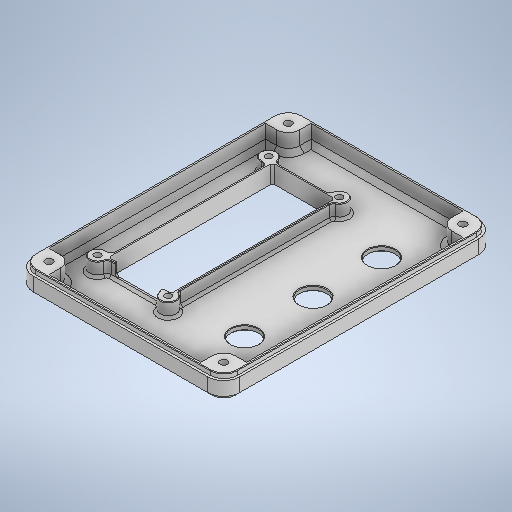
# Autodesk Inventor part: PCB-HousingBottom
Saved by Autodesk Inventor 2025.1 (Build 291241000, 241)
## iProperties
Created: 2025-03-29
Part Number: PCB-HousingBottom
Material: Všeobecné
Document SubType Name: Modeling
Designer: 42060
Density: 1 g/cm^3
Appearance: Výchozí
Author: 42060
Autodesk Inventor part; units mm, degrees
(part 1 of 4)
ref_plane "YZ Plane" through (0, 0, 0) normal (1, 0, 0) x (0, 1, 0)
ref_plane "XZ Plane" through (0, 0, 0) normal (0, 1, 0) x (-1, 0, 0)
ref_plane "XY Plane" through (0, 0, 0) normal (0, 0, 1) x (1, 0, 0)
sketch "Náčrt1" plane through (0, 0, 0) normal (0, 1, 0) x (-1, 0, 0)
  circle A0 centre (37.7, 43.65) radius 1.6
  circle A1 centre (-19.7, 43.65) radius 1.6
  arc A2 (41.3, 43.65) -> (37.7, 47.25) centre (37.7, 43.65) ccw
  arc A3 (-19.7, 47.25) -> (-23.3, 43.65) centre (-19.7, 43.65) ccw
  line L0 (38.3, 57.45) -> (-38.3, 57.45)
  line L1 (37.7, 47.25) -> (-19.7, 47.25)
  line L2 (-43.3, 52.45) -> (-43.3, -52.45)
  line L3 (-43.3, 57.45) -> (43.3, -57.45) construction
  line L4 (43.3, 57.45) -> (-43.3, -57.45) construction
  line L5 (43.3, -52.45) -> (43.3, 52.45)
  line L6 (41.3, -43.65) -> (41.3, 43.65)
  line L7 (-23.3, 43.65) -> (-23.3, -43.65)
  line L8 (41.3, 47.25) -> (-23.3, -47.25) construction
  line L9 (-23.3, 47.25) -> (41.3, -47.25) construction
  line L10 (-38.3, -57.45) -> (38.3, -57.45)
  circle A4 centre (37.7, -43.65) radius 1.6
  arc A5 (37.7, -47.25) -> (41.3, -43.65) centre (37.7, -43.65) ccw
  circle A6 centre (-19.7, -43.65) radius 1.6
  line L11 (-19.7, -47.25) -> (37.7, -47.25)
  arc A7 (-23.3, -43.65) -> (-19.7, -47.25) centre (-19.7, -43.65) ccw
  arc A8 (43.3, 52.45) -> (38.3, 57.45) centre (38.3, 52.45) ccw
  arc A9 (38.3, -57.45) -> (43.3, -52.45) centre (38.3, -52.45) ccw
  arc A10 (-43.3, -52.45) -> (-38.3, -57.45) centre (-38.3, -52.45) ccw
  arc A11 (-38.3, 57.45) -> (-43.3, 52.45) centre (-38.3, 52.45) ccw
  line L12 (45.3, 52.45) -> (45.3, -52.45)
  arc A12 (38.3, -59.45) -> (45.3, -52.45) centre (38.3, -52.45) ccw
  line L13 (38.3, -59.45) -> (-38.3, -59.45)
  arc A13 (-45.3, -52.45) -> (-38.3, -59.45) centre (-38.3, -52.45) ccw
  line L14 (-45.3, -52.45) -> (-45.3, 52.45)
  arc A14 (-38.3, 59.45) -> (-45.3, 52.45) centre (-38.3, 52.45) ccw
  line L15 (-38.3, 59.45) -> (38.3, 59.45)
  arc A15 (45.3, 52.45) -> (38.3, 59.45) centre (38.3, 52.45) ccw
  circle A16 centre (-38.3, 52.45) radius 1.625
  circle A17 centre (-38.3, 52.45) radius 5
  line L16 (-38.3, 47.45) -> (-43.3, 47.45)
  line L17 (-33.3, 52.45) -> (-33.3, 57.45)
  line L18 (43.3, 0) -> (-43.3, 0)
  line L19 (0, 57.45) -> (0, -57.45)
  circle A18 centre (-38.3, -52.45) radius 1.625
  circle A19 centre (-38.3, -52.45) radius 5
  line L20 (-38.3, -47.45) -> (-43.3, -47.45)
  line L21 (-33.3, -52.45) -> (-33.3, -57.45)
  circle A20 centre (38.3, 52.45) radius 5
  circle A21 centre (38.3, 52.45) radius 1.625
  line L22 (33.3, 52.45) -> (33.3, 57.45)
  circle A22 centre (38.3, -52.45) radius 5
  circle A23 centre (38.3, -52.45) radius 1.625
  line L23 (33.3, -52.45) -> (33.3, -57.45)
  line L24 (38.3, -47.45) -> (43.3, -47.45)
  line L25 (38.3, 47.45) -> (43.3, 47.45)
  point P0 (0, 0)
  point P1 (0, 0)
  point P2 (0, 0)
  point P3 (-43.3, -47.45)
  point P4 (-33.3, -57.45)
  point P5 (39.783171, -46.586051)
  point P6 (39.099517, -45.78373)
  point P7 (39.783171, 49.186051)
  point P8 (39.099517, 45.78373)
  point P9 (43.3, -52.45)
  point P10 (38.3, -57.45)
  point P11 (43.3, -52.45)
  point P12 (38.3, -57.45)
  dimension "d0" = 94.5
  dimension "d1" = 64.6
  dimension "d2" = 3.2
  dimension "d3" = 3.6
  dimension "d4" = 3.6
  dimension "d5" = 3.6
  dimension "d6" = 3.6
  dimension "d7" = 3.6
  dimension "d10" = 2
  dimension "d11" = 10.2
  dimension "d12" = 20
  dimension "d13" = 10.2
  dimension "d14" = 5
  dimension "d15" = 2
  dimension "d59" = 3.25
  constraints: 52 end point, 32 point on circle, 24 centre point, 21 point on line, 21 tangent, 12 equal radius, 10 symmetric about line, 8 coincident, 6 midpoint, 6 parallel, 5 perpendicular, 4 horizontal, 2 horizontal alignment, 2 vertical alignment, 1 vertical, 11 other
  measures "d0" distance of L9.end L8.start
  measures "d1" distance of L8.end L9.end
  measures "d2" diameter of A0
  measures "d3" distance from line of L6 A0.centre
  measures "d4" distance from line of L1 A0.centre
  measures "d5" distance from line of L7 A1.centre
  measures "d6" distance from line of L11 A4.centre
  measures "d7" radius of A3
  measures "d10" distance between parallel lines of L5 L6
  measures "d11" distance between parallel lines of L10 L11
  measures "d12" distance between parallel lines of L2 L7
  measures "d13" distance between parallel lines of L0 L1
  measures "d14" radius of A8
  measures "d15" distance between parallel lines of L5 L12
  measures "d59" diameter of A16
extrude "Vysunutí1" add sketch "Náčrt1" against normal blind 2 contours A0 | A1 | L6 L18 L19 L1 A2 | A2 L1 L19 L0 L22 A20 L25 L5 L18 L6 | L18 L5 L24 A22 L23 L10 L19 L11 A5 L6 | L6 A5 L11 L19 L18 | L19 L18 L7 A3 L1 | L1 A3 L7 L18 L2 L16 A17 L17 L0 L19 | L19 L11 A7 L7 L18 | L5 A22 L24 | L25 A20 L5 | L7 A7 L11 L19 L10 L21 A19 L20 L2 L18 | L0 A20 L22 | L17 A17 L0 | A9 A22 | A20 A8 | A17 A11 | L10 L23 A22 | L2 A17 L16 | L20 A19 L2 | L10 A19 L21 | A19 A10 | A4 | A6 | L12 A12 L13 A13 L14 A14 L15 A15
extrude "Vysunutí2" add sketch "Náčrt1" along normal blind 8 contours L5 A22 L24 | L25 A20 L5 | L0 A20 L22 | L17 A17 L0 | A9 A22 | A20 A8 | A17 A11 | L10 L23 A22 | L2 A17 L16 | L20 A19 L2 | L10 A19 L21 | A19 A10 | L12 A12 L13 A13 L14 A14 L15 A15
sketch "Náčrt2" plane through (0, 0, 0) normal (0, -1, 0) x (1, 0, 0)
  circle A0 centre (25, -30) radius 6
  circle A1 centre (25, 0) radius 6
  circle A2 centre (25, 30) radius 6
  line L0 (-28.4, -35.65) -> (-1.6, -35.65)
  line L1 (-1.6, -35.65) -> (-1.6, 35.65)
  line L2 (-1.6, 35.65) -> (-28.4, 35.65)
  line L3 (-28.4, 35.65) -> (-28.4, -35.65)
  line L4 (-28.4, -35.65) -> (-1.6, 35.65) construction
  line L5 (-1.6, -35.65) -> (-28.4, 35.65) construction
  line L6 (25, -30) -> (25, 0) construction
  line L7 (25, 0) -> (25, 30) construction
  circle A3 centre (-32, 37.5) radius 1.45
  circle A4 centre (-32, -37.5) radius 1.45
  circle A5 centre (-1, -37.5) radius 1.45
  circle A6 centre (-1, 37.5) radius 1.45
  line L8 (-28.7, -35.95) -> (-1.3, -35.95)
  line L9 (-1.3, -35.95) -> (-1.3, 35.95)
  line L10 (-1.3, 35.95) -> (-28.7, 35.95)
  line L11 (-28.7, 35.95) -> (-28.7, -35.95)
  arc A7 (-31.681818, -34.014493) -> (-28.591591, -38.295455) centre (-32, -37.5) ccw
  arc A8 (-28.591591, 38.295455) -> (-31.681818, 34.014493) centre (-32, 37.5) ccw
  line L12 (-6.356071, -36.75) -> (-26.643929, -36.75)
  line L13 (-29.5, -32.022774) -> (-29.5, 32.022774)
  line L14 (-26.643929, 36.75) -> (-6.356071, 36.75)
  line L15 (-0.5, 32.601021) -> (-0.5, -32.601021)
  arc A9 (-4.408409, -38.295455) -> (-6.356071, -36.75) centre (-6.356071, -38.75) ccw
  arc A10 (-0.5, -32.601021) -> (0.590909, -34.382468) centre (1.5, -32.601021) ccw
  arc A11 (0.590909, 34.382468) -> (-0.5, 32.601021) centre (1.5, 32.601021) ccw
  arc A12 (-6.356071, 36.75) -> (-4.408409, 38.295455) centre (-6.356071, 38.75) ccw
  arc A13 (-28.591591, 38.295455) -> (-26.643929, 36.75) centre (-26.643929, 38.75) ccw
  arc A14 (-29.5, 32.022774) -> (-31.681818, 34.014493) centre (-31.5, 32.022774) ccw
  arc A15 (-31.681818, -34.014493) -> (-29.5, -32.022774) centre (-31.5, -32.022774) ccw
  arc A16 (-26.643929, -36.75) -> (-28.591591, -38.295455) centre (-26.643929, -38.75) ccw
  arc A17 (-4.408409, -38.295455) -> (0.590909, -34.382468) centre (-1, -37.5) ccw
  arc A18 (0.590909, 34.382468) -> (-4.408409, 38.295455) centre (-1, 37.5) ccw
  line L16 (-29.5, -33.25) -> (-28.4, -33.25)
  arc A19 (-29.5, -33.25) -> (-30.15522, -33.503169) centre (-29.5, -34.224465) ccw
  line L17 (-29.5, 7.3) -> (-28.4, 7.3)
  line L18 (-25, 36.75) -> (-25, 35.65)
  line L19 (-5, 36.75) -> (-5, 35.65)
  arc A20 (-4.73177, 37.583104) -> (-5, 36.75) centre (-3.572102, 36.75) ccw
  point P0 (0, 0)
  point P1 (-15, 0)
  point P2 (-28.7, -33.25)
  point P3 (-28.7, 7.3)
  point P4 (-15, 35.65)
  point P5 (-5, 35.95)
  point P6 (-25, 35.95)
  dimension "d23" = 71.3
  dimension "d24" = 26.8
  dimension "d25" = 12
  dimension "d26" = 2.9
  dimension "d27" = 75
  dimension "d28" = 31
  dimension "d30" = 1.85
  dimension "d31" = 3.6
  dimension "d32" = 0.3
  dimension "d33" = 30
  dimension "d34" = 15
  dimension "d35" = 25
  dimension "d39" = 0.8
  dimension "d40" = 0.8
  dimension "d41" = 0.8
  dimension "d42" = 0.8
  dimension "d43" = 2
  dimension "d44" = 3.5
  dimension "d47" = 2.4
  dimension "d48" = 40.55
  dimension "d49" = 10
  dimension "d50" = 20
  constraints: 40 end point, 30 point on circle, 21 centre point, 20 tangent, 15 equal radius, 8 point on line, 6 parallel, 6 perpendicular, 4 coincident, 4 horizontal alignment, 4 vertical alignment, 3 horizontal, 3 midpoint, 2 collinear, 1 vertical, 3 other
  measures "d23" distance of L2.end L0.start
  measures "d24" distance between parallel lines of L1 L3
  measures "d25" diameter of A0
  measures "d26" diameter of A3
  measures "d27" distance of A4.centre A3.centre
  measures "d28" distance of A6.centre A3.centre
  measures "d30" distance from line of A3.centre L2
  measures "d31" distance from line of L3 A3.centre
  measures "d32" distance between parallel lines of L3 L11
  measures "d33" distance of L6.end L7.end
  measures "d34" distance of point (0, 0) point (-15, 0)
  measures "d35" distance of L6.end point (0, 0)
  measures "d39" distance between parallel lines of L8 L12
  measures "d40" distance between parallel lines of L11 L13
  measures "d41" distance between parallel lines of L10 L14
  measures "d42" distance between parallel lines of L9 L15
  measures "d43" radius of A9
  measures "d44" radius of A17
  measures "d47" distance between parallel lines of L0 L16
  measures "d48" distance between parallel lines of L16 L17
  measures "d49" distance from line of point (-15, 35.65) L18
  measures "d50" distance between parallel lines of L19 L18
extrude "Vysunutí4" cut sketch "Náčrt2" along normal through all contours A0 | A1 | A2 | L3 L2 L1 L0 | L0 L1 L2 L19 L10 L9 L8 L11 L16 L3 | L16 L11 L17 L3 | L17 L11 L10 L18 L2 L3 | L2 L18 L10 L19
extrude "Vysunutí5" add sketch "Náčrt2" against normal blind 6.1 contours L16 A19 A15 L13 L17 L11 | L11 L8 L9 L10 L19 A20 A12 A18 A11 L15 A10 A17 A9 L12 A16 A7 A15 A19 L16 | L17 L13 A14 A8 A13 L14 L18 L10 L11
extrude "Vysunutí6" add sketch "Náčrt2" against normal blind 1 contours L10 L18 L14 A12 A20 L19
chamfer "Zkosení1" distance 1 angle 45 3 edges at (-25, 1, 36.35) (-5, 1, 36.35) (-4.9313, 1, 37.1876)
sketch "Náčrt3" plane through (0, 8, 0) normal (0, 1, 0) x (1, 0, 0)
  line L0 (45.3, -52.45) -> (45.3, 52.45) projected
  arc A0 (45.3, 52.45) -> (38.3, 59.45) centre (38.3, 52.45) ccw projected
  line L1 (38.3, 59.45) -> (-38.3, 59.45) projected
  arc A1 (-38.3, 59.45) -> (-45.3, 52.45) centre (-38.3, 52.45) ccw projected
  line L2 (-45.3, 52.45) -> (-45.3, -52.45) projected
  arc A2 (-45.3, -52.45) -> (-38.3, -59.45) centre (-38.3, -52.45) ccw projected
  line L3 (-38.3, -59.45) -> (38.3, -59.45) projected
  arc A3 (38.3, -59.45) -> (45.3, -52.45) centre (38.3, -52.45) ccw projected
  line L4 (-33.3, 57.45) -> (33.3, 57.45) projected
  line L5 (43.3, 47.45) -> (43.3, -47.45) projected
  line L6 (33.3, -57.45) -> (-33.3, -57.45) projected
  line L7 (-43.3, -47.45) -> (-43.3, 47.45) projected
  line L8 (33.3, 57.45) -> (33.3, 52.45) projected
  arc A4 (33.3, 52.45) -> (38.3, 47.45) centre (38.3, 52.45) ccw projected
  line L9 (38.3, 47.45) -> (43.3, 47.45) projected
  line L10 (43.3, -47.45) -> (38.3, -47.45) projected
  arc A5 (38.3, -47.45) -> (33.3, -52.45) centre (38.3, -52.45) ccw projected
  line L11 (33.3, -52.45) -> (33.3, -57.45) projected
  line L12 (-38.3, 58.4) -> (38.3, 58.4)
  arc A6 (44.25, 52.45) -> (38.3, 58.4) centre (38.3, 52.45) ccw
  line L13 (44.25, 52.45) -> (44.25, -52.45)
  arc A7 (38.3, -58.4) -> (44.25, -52.45) centre (38.3, -52.45) ccw
  line L14 (38.3, -58.4) -> (-38.3, -58.4)
  arc A8 (-44.25, -52.45) -> (-38.3, -58.4) centre (-38.3, -52.45) ccw
  line L15 (-44.25, -52.45) -> (-44.25, 52.45)
  arc A9 (-38.3, 58.4) -> (-44.25, 52.45) centre (-38.3, 52.45) ccw
  line L16 (-43.3, 47.45) -> (-38.3, 47.45) projected
  arc A10 (-38.3, 47.45) -> (-33.3, 52.45) centre (-38.3, 52.45) ccw projected
  line L17 (-33.3, 52.45) -> (-33.3, 57.45) projected
  line L18 (-33.3, -57.45) -> (-33.3, -52.45) projected
  arc A11 (-33.3, -52.45) -> (-38.3, -47.45) centre (-38.3, -52.45) ccw projected
  line L19 (-38.3, -47.45) -> (-43.3, -47.45) projected
  point P0 (0, 0)
  dimension "d67" = 1.05
  constraints: 8 end point, 8 point on circle, 4 centre point, 7 other
  measures "d67" distance between parallel lines of L1 L12
extrude "Vysunutí7" cut sketch "Náčrt3" against normal blind 2 contours A3 L3 A2 L2 A1 L1 A0 L0
sketch "Náčrt4" plane through (0, -2, 0) normal (0, -1, 0) x (1, 0, 0)
  circle A0 centre (-38.3, -52.45) radius 1.625 projected
  circle A1 centre (-38.3, 52.45) radius 1.625 projected
  circle A2 centre (38.3, 52.45) radius 1.625 projected
  circle A3 centre (38.3, -52.45) radius 1.625 projected
  point P0 (0, 0)
  constraints: 4 coincident
hole "Díra1" at (-38.3, -2, -52.45) at (-38.3, -2, 52.45) at (38.3, -2, 52.45) at (38.3, -2, -52.45) direction (0, 1, 0) diameter 5.7 depth 3
chamfer "Zkosení3" distance 2 angle 45 24 edges at (34.7645, 0, -48.9145) (33.3, 0, -54.95) (40.8, 0, -47.45) (43.3, 0, 0) (33.3, 0, 54.95) (34.7645, 0, 48.9145) (40.8, 0, 47.45) (0, 0, 57.45) (-34.7645, 0, 48.9145) (-33.3, 0, 54.95) (-40.8, 0, 47.45) (-43.3, 0, 0) (-33.3, 0, -54.95) (-34.7645, 0, -48.9145) (-40.8, 0, -47.45) (0, 0, -57.45) (0, -2, -59.45) (43.2497, -2, -57.3997) (45.3, -2, 0) (43.2497, -2, 57.3997) (0, -2, 59.45) (-43.2497, -2, 57.3997) (-45.3, -2, 0) (-43.2497, -2, -57.3997)
chamfer "Zkosení5" distance 1 angle 45 20 edges at (-1.3, 2.05, 35.95) (-1.3, 2.05, -35.95) (-28.7, 2.05, -35.95) (-28.7, 2.05, 35.95) (-16.5, 0, 36.75) (-27.8871, 0, 37.1833) (-34.8379, 0, 39.5485) (-30.1516, 0, 33.4999) (-29.5, 0, 0) (-30.1516, 0, -33.4999) (-34.8379, 0, -39.5485) (-27.8871, 0, -37.1833) (-16.5, 0, -36.75) (-5.1129, 0, -37.1833) (1.1572, 0, -40.2561) (-0.2056, 0, -33.6455) (-0.5, 0, 0) (-0.2056, 0, 33.6455) (1.1572, 0, 40.2561) (-5.1129, 0, 37.1833)
chamfer "Zkosení2" distance 0.25 angle 45 44 edges at (-44.25, 8, 0) (-42.5073, 8, 56.6573) (0, 8, 58.4) (42.5073, 8, 56.6573) (44.25, 8, 0) (42.5073, 8, -56.6573) (0, 8, -58.4) (-42.5073, 8, -56.6573) (19, 0, -30) (19, -2, -30) (19, 0, 0) (19, -2, 0) (19, 0, 30) (19, -2, 30) (-1.3, -2, 0) (-15, -2, -35.95) (-28.7, -2, 0) (-15, -2, 35.95) (38.3, -2, 55.3) (38.3, -2, -49.6) (-38.3, -2, -49.6) (-38.3, -2, 55.3) (-27.8871, 6.1, 37.1833) (-25.822, 6.1, 36.75) (-34.8379, 6.1, 39.5485) (-30.1516, 6.1, 33.4999) (-29.5, 6.1, 0) (-30.1516, 6.1, -33.4999) (-34.8379, 6.1, -39.5485) (-27.8871, 6.1, -37.1833) (-16.5, 6.1, -36.75) (-5.1129, 6.1, -37.1833) (1.1572, 6.1, -40.2561) (-0.2056, 6.1, -33.6455) (-0.5, 6.1, 0) (-0.2056, 6.1, 33.6455) (1.1572, 6.1, 40.2561) (-4.5349, 6.1, 37.9233) (-4.9313, 6.1, 37.1876) (-5, 6.1, 36.35) (-28.2001, -2, -35.45) (-28.2, -2, 35.45) (-1.8, -2, 35.4501) (-1.8, -2, -35.45)
sketch "Náčrt5" plane through (0, -2, 0) normal (0, -1, 0) x (1, 0, 0)
  line L0 (3.529017, -37.317035) -> (3.529017, -22.682965) construction
  line L1 (3.529017, -22.682965) -> (6.470983, -22.682965) construction
  line L2 (6.470983, -22.682965) -> (6.470983, -37.317035) construction
  line L3 (6.470983, -37.317035) -> (3.529017, -37.317035) construction
  line L4 (3.529017, -8.753762) -> (3.529017, 8.753762) construction
  line L5 (3.529017, 8.753762) -> (6.470983, 8.753762) construction
  line L6 (6.470983, 8.753762) -> (6.470983, -8.753762) construction
  line L7 (6.470983, -8.753762) -> (3.529017, -8.753762) construction
  line L8 (3.529017, 19.285961) -> (3.529017, 40.714039) construction
  line L9 (3.529017, 40.714039) -> (6.470983, 40.714039) construction
  line L10 (6.470983, 40.714039) -> (6.470983, 19.285961) construction
  line L11 (6.470983, 19.285961) -> (3.529017, 19.285961) construction
  circle A0 centre (25, -30) radius 6.25
  circle A1 centre (25, 0) radius 6.25
  circle A2 centre (25, 30) radius 6.25
  line L12 (-40.028603, -44.09129) -> (-40.028603, 44.09129) construction
  line L13 (-40.028603, 44.09129) -> (-36.91312, 44.09129) construction
  line L14 (-36.91312, 44.09129) -> (-36.91312, -44.09129) construction
  line L15 (-36.91312, -44.09129) -> (-40.028603, -44.09129) construction
  line L16 (-43.3, -52.45) -> (-43.3, 52.45)
  line L17 (3.534054, -35.342469) -> (3.534054, -34.612081)
  line L18 (3.534054, -34.612081) -> (9.634054, -32.748332)
  line L19 (9.634054, -32.748332) -> (9.634054, -33.760801)
  line L20 (9.634054, -33.760801) -> (5.150982, -34.974756)
  line L21 (5.150982, -34.974756) -> (9.634054, -36.188712)
  line L22 (9.634054, -36.188712) -> (9.634054, -37.206218)
  line L23 (9.634054, -37.206218) -> (3.534054, -35.342469)
  line L24 (7.573856, -36.188712) -> (7.573856, -33.715466)
  line L25 (7.573856, -33.715466) -> (8.485582, -33.715466)
  line L26 (8.485582, -33.715466) -> (8.485582, -36.188712)
  line L27 (8.485582, -36.188712) -> (7.573856, -36.188712)
  line L28 (6.163451, -31.660305) -> (6.163451, -30.053451)
  spline S0 degree 2 poles (6.163451, -30.053451) (6.163451, -29.857002) (6.002262, -29.574921) (5.689958, -29.418769) (5.478397, -29.418769) knots 0 0 0 1 2 3 3 3
  line L29 (5.478397, -29.418769) -> (5.150982, -29.418769)
  spline S1 degree 2 poles (5.150982, -29.418769) (4.939421, -29.418769) (4.62208, -29.574921) (4.44578, -29.857002) (4.44578, -30.053451) knots 0 0 0 1 2 3 3 3
  line L30 (4.44578, -30.053451) -> (4.44578, -31.660305)
  line L31 (4.44578, -31.660305) -> (3.529017, -31.660305)
  line L32 (3.529017, -31.660305) -> (3.529017, -30.0736)
  spline S2 degree 2 poles (3.529017, -30.0736) (3.529017, -29.569884) (3.911841, -28.824385) (4.632155, -28.426449) (5.120759, -28.426449) knots 0 0 0 1 2 3 3 3
  line L33 (5.120759, -28.426449) -> (5.47336, -28.426449)
  spline S3 degree 2 poles (5.47336, -28.426449) (5.967002, -28.426449) (6.692353, -28.824385) (7.085251, -29.569884) (7.085251, -30.0736) knots 0 0 0 1 2 3 3 3
  line L34 (7.085251, -30.0736) -> (7.085251, -31.660305)
  line L35 (7.085251, -31.660305) -> (6.163451, -31.660305)
  line L36 (3.529017, -32.07839) -> (3.529017, -31.121329)
  line L37 (3.529017, -31.121329) -> (9.634054, -31.121329)
  line L38 (9.634054, -31.121329) -> (9.634054, -32.07839)
  line L39 (9.634054, -32.07839) -> (3.529017, -32.07839)
  line L40 (6.893839, -30.451387) -> (6.702427, -29.504401)
  line L41 (6.702427, -29.504401) -> (9.634054, -28.214888)
  line L42 (9.634054, -28.214888) -> (9.634054, -29.312989)
  line L43 (9.634054, -29.312989) -> (6.893839, -30.451387)
  line L44 (9.719474, -22.556254) -> (9.719474, -23.249664)
  line L45 (9.719474, -23.249664) -> (5.036443, -23.249664)
  line L46 (5.036443, -23.249664) -> (8.242209, -24.852547)
  line L47 (8.242209, -24.852547) -> (5.036443, -26.45543)
  line L48 (5.036443, -26.45543) -> (9.719474, -26.45543)
  line L49 (9.719474, -26.45543) -> (9.719474, -27.14884)
  line L50 (9.719474, -27.14884) -> (3.619474, -27.14884)
  line L51 (3.619474, -27.14884) -> (3.619474, -26.555924)
  line L52 (3.619474, -26.555924) -> (6.955883, -24.852547)
  line L53 (6.955883, -24.852547) -> (3.619474, -23.149169)
  line L54 (3.619474, -23.149169) -> (3.619474, -22.556254)
  line L55 (3.619474, -22.556254) -> (9.719474, -22.556254)
  spline S4 degree 2 poles (9.754946, -6.537412) (9.754946, -7.03609) (9.457753, -7.806776) (8.868405, -8.315529) (8.43521, -8.416272) knots 0 0 0 1 2 3 3 3
  line L56 (8.43521, -8.416272) -> (8.037274, -7.509583)
  spline S5 degree 2 poles (8.037274, -7.509583) (8.425135, -7.398766) (8.828108, -6.879939) (8.828108, -6.502152) knots 0 0 0 1 2 2 2
  spline S6 degree 2 poles (8.828108, -6.502152) (8.828108, -6.07903) (8.455358, -5.605537) (8.122906, -5.605537) knots 0 0 0 1 2 2 2
  line L57 (8.122906, -5.605537) -> (7.850899, -5.605537)
  spline S7 degree 2 poles (7.850899, -5.605537) (7.614153, -5.605537) (7.306886, -5.867469) (7.135623, -6.270442) (7.034879, -6.602895) knots 0 0 0 1 2 3 3 3
  spline S8 degree 2 poles (7.034879, -6.602895) (7.029842, -6.607932) (7.024805, -6.628081) (7.019768, -6.638155) knots 0 0 0 1 2 2 2
  line L58 (7.019768, -6.638155) -> (7.009694, -6.683489)
  spline S9 degree 2 poles (7.009694, -6.683489) (6.863616, -7.187205) (6.556349, -7.821887) (5.896481, -8.270195) (5.337357, -8.270195) knots 0 0 0 1 2 3 3 3
  line L59 (5.337357, -8.270195) -> (5.17113, -8.270195)
  spline S10 degree 2 poles (5.17113, -8.270195) (4.652303, -8.270195) (3.911841, -7.836999) (3.529016, -7.005868) (3.529016, -6.421557) knots 0 0 0 1 2 3 3 3
  spline S11 degree 2 poles (3.529016, -6.421557) (3.529016, -5.978287) (3.821172, -5.29827) (4.385334, -4.839889) (4.803418, -4.729071) knots 0 0 0 1 2 3 3 3
  line L60 (4.803418, -4.729071) -> (5.206391, -5.6005)
  spline S12 degree 2 poles (5.206391, -5.6005) (4.838678, -5.711318) (4.455854, -6.154588) (4.455854, -6.45178) knots 0 0 0 1 2 2 2
  spline S13 degree 2 poles (4.455854, -6.45178) (4.455854, -6.864827) (4.808455, -7.313134) (5.130833, -7.313134) knots 0 0 0 1 2 2 2
  line L61 (5.130833, -7.313134) -> (5.33232, -7.313134)
  spline S14 degree 2 poles (5.33232, -7.313134) (5.584178, -7.313134) (5.891444, -7.046165) (6.067745, -6.638155) (6.173525, -6.280517) knots 0 0 0 1 2 3 3 3
  spline S15 degree 2 poles (6.173525, -6.280517) (6.183599, -6.260368) (6.193674, -6.220071) (6.203748, -6.194885) knots 0 0 0 1 2 2 2
  spline S16 degree 2 poles (6.203748, -6.194885) (6.208785, -6.179773) (6.21886, -6.139476) (6.223897, -6.119327) knots 0 0 0 1 2 2 2
  spline S17 degree 2 poles (6.223897, -6.119327) (6.364937, -5.660946) (6.682278, -5.061524) (7.31696, -4.653514) (7.845862, -4.653514) knots 0 0 0 1 2 3 3 3
  line L62 (7.845862, -4.653514) -> (8.117869, -4.653514)
  spline S18 degree 2 poles (8.117869, -4.653514) (8.636696, -4.653514) (9.372121, -5.096784) (9.754946, -5.943027) (9.754946, -6.537412) knots 0 0 0 1 2 3 3 3
  line L63 (4.098215, -2.961028) -> (4.098215, -1.998931)
  line L64 (4.098215, -1.998931) -> (9.6945, -1.998931)
  line L65 (9.6945, -1.998931) -> (9.6945, -2.961028)
  line L66 (9.6945, -2.961028) -> (4.098215, -2.961028)
  line L67 (3.5945, -4.331136) -> (3.5945, -0.628824)
  line L68 (3.5945, -0.628824) -> (4.511263, -0.628824)
  line L69 (4.511263, -0.628824) -> (4.511263, -4.331136)
  line L70 (4.511263, -4.331136) -> (3.5945, -4.331136)
  spline S19 degree 2 poles (9.754946, 1.647973) (9.754946, 1.083811) (9.306638, 0.237568) (8.460396, -0.215777) (7.891197, -0.215777) knots 0 0 0 1 2 3 3 3
  line L71 (7.891197, -0.215777) -> (5.397803, -0.215777)
  spline S20 degree 2 poles (5.397803, -0.215777) (4.828604, -0.215777) (3.982361, 0.237568) (3.529016, 1.083811) (3.529016, 1.647973) knots 0 0 0 1 2 3 3 3
  spline S21 degree 2 poles (3.529016, 1.647973) (3.529016, 2.217172) (3.982361, 3.058377) (4.828604, 3.511722) (5.397803, 3.511722) knots 0 0 0 1 2 3 3 3
  line L72 (5.397803, 3.511722) -> (7.891197, 3.511722)
  spline S22 degree 2 poles (7.891197, 3.511722) (8.460396, 3.511722) (9.306638, 3.058377) (9.754946, 2.217172) (9.754946, 1.647973) knots 0 0 0 1 2 3 3 3
  spline S23 degree 2 poles (8.802922, 1.647973) (8.802922, 1.919979) (8.57625, 2.317915) (8.158166, 2.529475) (7.876085, 2.529475) knots 0 0 0 1 2 3 3 3
  line L73 (7.876085, 2.529475) -> (5.407877, 2.529475)
  spline S24 degree 2 poles (5.407877, 2.529475) (5.125796, 2.529475) (4.707712, 2.317915) (4.48104, 1.919979) (4.48104, 1.647973) knots 0 0 0 1 2 3 3 3
  spline S25 degree 2 poles (4.48104, 1.647973) (4.48104, 1.381003) (4.707712, 0.983067) (5.125796, 0.76647) (5.407877, 0.76647) knots 0 0 0 1 2 3 3 3
  line L74 (5.407877, 0.76647) -> (7.876085, 0.76647)
  spline S26 degree 2 poles (7.876085, 0.76647) (8.158166, 0.76647) (8.57625, 0.983067) (8.802922, 1.381003) (8.802922, 1.647973) knots 0 0 0 1 2 3 3 3
  line L75 (6.410272, 5.032944) -> (6.410272, 6.569277)
  spline S27 degree 2 poles (6.410272, 6.569277) (6.410272, 6.760689) (6.228934, 7.052845) (5.896481, 7.208997) (5.674846, 7.208997) knots 0 0 0 1 2 3 3 3
  line L76 (5.674846, 7.208997) -> (5.261799, 7.208997)
  spline S28 degree 2 poles (5.261799, 7.208997) (5.035127, 7.208997) (4.6926, 7.052845) (4.511263, 6.760689) (4.511263, 6.569277) knots 0 0 0 1 2 3 3 3
  line L77 (4.511263, 6.569277) -> (4.511263, 5.032944)
  line L78 (4.511263, 5.032944) -> (3.5945, 5.032944)
  line L79 (3.5945, 5.032944) -> (3.5945, 6.554166)
  spline S29 degree 2 poles (3.5945, 6.554166) (3.5945, 7.057882) (3.987398, 7.793307) (4.722823, 8.191243) (5.221502, 8.191243) knots 0 0 0 1 2 3 3 3
  line L80 (5.221502, 8.191243) -> (5.720181, 8.191243)
  spline S30 degree 2 poles (5.720181, 8.191243) (6.213822, 8.191243) (6.939173, 7.793307) (7.327035, 7.057882) (7.327035, 6.554166) knots 0 0 0 1 2 3 3 3
  line L81 (7.327035, 6.554166) -> (7.327035, 5.032944)
  line L82 (7.327035, 5.032944) -> (6.410272, 5.032944)
  line L83 (3.5945, 4.559451) -> (3.5945, 5.521548)
  line L84 (3.5945, 5.521548) -> (9.6945, 5.521548)
  line L85 (9.6945, 5.521548) -> (9.6945, 4.559451)
  line L86 (9.6945, 4.559451) -> (3.5945, 4.559451)
  line L87 (6.223897, 20.258133) -> (6.223897, 21.864987)
  spline S31 degree 2 poles (6.223897, 21.864987) (6.223897, 22.061436) (6.062708, 22.343517) (5.750404, 22.499669) (5.538843, 22.499669) knots 0 0 0 1 2 3 3 3
  line L88 (5.538843, 22.499669) -> (5.211428, 22.499669)
  spline S32 degree 2 poles (5.211428, 22.499669) (4.999867, 22.499669) (4.682526, 22.343517) (4.506225, 22.061436) (4.506225, 21.864987) knots 0 0 0 1 2 3 3 3
  line L89 (4.506225, 21.864987) -> (4.506225, 20.258133)
  line L90 (4.506225, 20.258133) -> (3.589462, 20.258133)
  line L91 (3.589462, 20.258133) -> (3.589462, 21.844838)
  spline S33 degree 2 poles (3.589462, 21.844838) (3.589462, 22.348554) (3.972286, 23.094054) (4.6926, 23.491989) (5.181205, 23.491989) knots 0 0 0 1 2 3 3 3
  line L92 (5.181205, 23.491989) -> (5.533806, 23.491989)
  spline S34 degree 2 poles (5.533806, 23.491989) (6.027448, 23.491989) (6.752799, 23.094054) (7.145697, 22.348554) (7.145697, 21.844838) knots 0 0 0 1 2 3 3 3
  line L93 (7.145697, 21.844838) -> (7.145697, 20.258133)
  line L94 (7.145697, 20.258133) -> (6.223897, 20.258133)
  line L95 (3.589462, 19.840049) -> (3.589462, 20.797109)
  line L96 (3.589462, 20.797109) -> (9.6945, 20.797109)
  line L97 (9.6945, 20.797109) -> (9.6945, 19.840049)
  line L98 (9.6945, 19.840049) -> (3.589462, 19.840049)
  line L99 (6.954285, 21.467051) -> (6.762873, 22.414037)
  line L100 (6.762873, 22.414037) -> (9.6945, 23.70355)
  line L101 (9.6945, 23.70355) -> (9.6945, 22.605449)
  line L102 (9.6945, 22.605449) -> (6.954285, 21.467051)
  line L103 (3.5945, 24.585053) -> (3.5945, 25.54715)
  line L104 (3.5945, 25.54715) -> (9.6945, 25.54715)
  line L105 (9.6945, 25.54715) -> (9.6945, 24.585053)
  line L106 (9.6945, 24.585053) -> (3.5945, 24.585053)
  line L107 (3.5945, 25.013211) -> (3.5945, 27.919652)
  line L108 (3.5945, 27.919652) -> (4.5163, 27.919652)
  line L109 (4.5163, 27.919652) -> (4.5163, 25.013211)
  line L110 (4.5163, 25.013211) -> (3.5945, 25.013211)
  line L111 (8.772699, 25.013211) -> (8.772699, 27.919652)
  line L112 (8.772699, 27.919652) -> (9.6945, 27.919652)
  line L113 (9.6945, 27.919652) -> (9.6945, 25.013211)
  line L114 (9.6945, 25.013211) -> (8.772699, 25.013211)
  line L115 (6.203748, 25.013211) -> (6.203748, 27.5872)
  line L116 (6.203748, 27.5872) -> (7.125548, 27.5872)
  line L117 (7.125548, 27.5872) -> (7.125548, 25.013211)
  line L118 (7.125548, 25.013211) -> (6.203748, 25.013211)
  spline S35 degree 2 poles (9.754946, 30.438232) (9.754946, 29.939553) (9.457753, 29.168868) (8.868405, 28.660115) (8.43521, 28.559372) knots 0 0 0 1 2 3 3 3
  line L119 (8.43521, 28.559372) -> (8.037274, 29.46606)
  spline S36 degree 2 poles (8.037274, 29.46606) (8.425135, 29.576878) (8.828108, 30.095705) (8.828108, 30.473492) knots 0 0 0 1 2 2 2
  spline S37 degree 2 poles (8.828108, 30.473492) (8.828108, 30.896614) (8.455358, 31.370107) (8.122906, 31.370107) knots 0 0 0 1 2 2 2
  line L120 (8.122906, 31.370107) -> (7.850899, 31.370107)
  spline S38 degree 2 poles (7.850899, 31.370107) (7.614153, 31.370107) (7.306886, 31.108174) (7.135623, 30.705202) (7.034879, 30.372749) knots 0 0 0 1 2 3 3 3
  spline S39 degree 2 poles (7.034879, 30.372749) (7.029842, 30.367712) (7.024805, 30.347563) (7.019768, 30.337489) knots 0 0 0 1 2 2 2
  line L121 (7.019768, 30.337489) -> (7.009694, 30.292154)
  spline S40 degree 2 poles (7.009694, 30.292154) (6.863616, 29.788439) (6.556349, 29.153756) (5.896481, 28.705449) (5.337357, 28.705449) knots 0 0 0 1 2 3 3 3
  line L122 (5.337357, 28.705449) -> (5.17113, 28.705449)
  spline S41 degree 2 poles (5.17113, 28.705449) (4.652303, 28.705449) (3.911841, 29.138645) (3.529016, 29.969776) (3.529016, 30.554087) knots 0 0 0 1 2 3 3 3
  spline S42 degree 2 poles (3.529016, 30.554087) (3.529016, 30.997357) (3.821172, 31.677373) (4.385334, 32.135755) (4.803418, 32.246572) knots 0 0 0 1 2 3 3 3
  line L123 (4.803418, 32.246572) -> (5.206391, 31.375144)
  spline S43 degree 2 poles (5.206391, 31.375144) (4.838678, 31.264326) (4.455854, 30.821056) (4.455854, 30.523864) knots 0 0 0 1 2 2 2
  spline S44 degree 2 poles (4.455854, 30.523864) (4.455854, 30.110817) (4.808455, 29.66251) (5.130833, 29.66251) knots 0 0 0 1 2 2 2
  line L124 (5.130833, 29.66251) -> (5.33232, 29.66251)
  spline S45 degree 2 poles (5.33232, 29.66251) (5.584178, 29.66251) (5.891444, 29.929479) (6.067745, 30.337489) (6.173525, 30.695127) knots 0 0 0 1 2 3 3 3
  spline S46 degree 2 poles (6.173525, 30.695127) (6.183599, 30.715276) (6.193674, 30.755573) (6.203748, 30.780759) knots 0 0 0 1 2 2 2
  spline S47 degree 2 poles (6.203748, 30.780759) (6.208785, 30.79587) (6.21886, 30.836168) (6.223897, 30.856316) knots 0 0 0 1 2 2 2
  spline S48 degree 2 poles (6.223897, 30.856316) (6.364937, 31.314698) (6.682278, 31.91412) (7.31696, 32.32213) (7.845862, 32.32213) knots 0 0 0 1 2 3 3 3
  line L125 (7.845862, 32.32213) -> (8.117869, 32.32213)
  spline S49 degree 2 poles (8.117869, 32.32213) (8.636696, 32.32213) (9.372121, 31.87886) (9.754946, 31.032617) (9.754946, 30.438232) knots 0 0 0 1 2 3 3 3
  line L126 (3.5945, 33.274153) -> (3.5945, 34.23625)
  line L127 (3.5945, 34.23625) -> (9.6945, 34.23625)
  line L128 (9.6945, 34.23625) -> (9.6945, 33.274153)
  line L129 (9.6945, 33.274153) -> (3.5945, 33.274153)
  line L130 (3.5945, 33.702311) -> (3.5945, 36.608752)
  line L131 (3.5945, 36.608752) -> (4.5163, 36.608752)
  line L132 (4.5163, 36.608752) -> (4.5163, 33.702311)
  line L133 (4.5163, 33.702311) -> (3.5945, 33.702311)
  line L134 (8.772699, 33.702311) -> (8.772699, 36.608752)
  line L135 (8.772699, 36.608752) -> (9.6945, 36.608752)
  line L136 (9.6945, 36.608752) -> (9.6945, 33.702311)
  line L137 (9.6945, 33.702311) -> (8.772699, 33.702311)
  line L138 (6.203748, 33.702311) -> (6.203748, 36.2763)
  line L139 (6.203748, 36.2763) -> (7.125548, 36.2763)
  line L140 (7.125548, 36.2763) -> (7.125548, 33.702311)
  line L141 (7.125548, 33.702311) -> (6.203748, 33.702311)
  line L142 (4.098215, 38.205532) -> (4.098215, 39.16763)
  line L143 (4.098215, 39.16763) -> (9.6945, 39.16763)
  line L144 (9.6945, 39.16763) -> (9.6945, 38.205532)
  line L145 (9.6945, 38.205532) -> (4.098215, 38.205532)
  line L146 (3.5945, 36.835425) -> (3.5945, 40.537737)
  line L147 (3.5945, 40.537737) -> (4.511263, 40.537737)
  line L148 (4.511263, 40.537737) -> (4.511263, 36.835425)
  line L149 (4.511263, 36.835425) -> (3.5945, 36.835425)
  line L150 (-39.974928, -43.504997) -> (-39.974928, -42.683362)
  line L151 (-39.974928, -42.683362) -> (-34.974928, -42.683362)
  line L152 (-34.974928, -42.683362) -> (-34.974928, -43.504997)
  line L153 (-34.974928, -43.504997) -> (-39.974928, -43.504997)
  line L154 (-35.763533, -43.121017) -> (-35.763533, -40.226715)
  line L155 (-35.763533, -40.226715) -> (-34.974928, -40.226715)
  line L156 (-34.974928, -40.226715) -> (-34.974928, -43.121017)
  line L157 (-34.974928, -43.121017) -> (-35.763533, -43.121017)
  line L158 (-34.974928, -38.661892) -> (-34.974928, -39.504171)
  line L159 (-34.974928, -39.504171) -> (-39.974928, -39.504171)
  line L160 (-39.974928, -39.504171) -> (-39.974928, -38.661892)
  line L161 (-39.974928, -38.661892) -> (-34.974928, -38.661892)
  line L162 (-34.921386, -33.742908) -> (-34.921386, -34.21243)
  line L163 (-34.921386, -34.21243) -> (-38.916444, -36.938954)
  line L164 (-38.916444, -36.938954) -> (-34.921386, -36.938954)
  line L165 (-34.921386, -36.938954) -> (-34.921386, -37.507323)
  line L166 (-34.921386, -37.507323) -> (-39.859607, -37.507323)
  line L167 (-39.859607, -37.507323) -> (-39.871963, -37.041919)
  line L168 (-39.871963, -37.041919) -> (-35.876905, -34.311277)
  line L169 (-35.876905, -34.311277) -> (-39.871963, -34.311277)
  line L170 (-39.871963, -34.311277) -> (-39.871963, -33.742908)
  line L171 (-39.871963, -33.742908) -> (-34.921386, -33.742908)
  line L172 (-39.974928, -32.687093) -> (-39.974928, -31.865458)
  line L173 (-39.974928, -31.865458) -> (-34.974928, -31.865458)
  line L174 (-34.974928, -31.865458) -> (-34.974928, -32.687093)
  line L175 (-34.974928, -32.687093) -> (-39.974928, -32.687093)
  line L176 (-39.974928, -32.34853) -> (-39.974928, -29.408811)
  line L177 (-39.974928, -29.408811) -> (-39.186324, -29.408811)
  line L178 (-39.186324, -29.408811) -> (-39.186324, -32.34853)
  line L179 (-39.186324, -32.34853) -> (-39.974928, -32.34853)
  line L180 (-35.763533, -32.34853) -> (-35.763533, -29.408811)
  line L181 (-35.763533, -29.408811) -> (-34.974928, -29.408811)
  line L182 (-34.974928, -29.408811) -> (-34.974928, -32.34853)
  line L183 (-34.974928, -32.34853) -> (-35.763533, -32.34853)
  line L184 (-37.852715, -32.34853) -> (-37.852715, -29.784533)
  line L185 (-37.852715, -29.784533) -> (-37.064111, -29.784533)
  line L186 (-37.064111, -29.784533) -> (-37.064111, -32.34853)
  line L187 (-37.064111, -32.34853) -> (-37.852715, -32.34853)
  line L188 (-39.974928, -26.584699) -> (-39.974928, -25.763064)
  line L189 (-39.974928, -25.763064) -> (-34.974928, -25.763064)
  line L190 (-34.974928, -25.763064) -> (-34.974928, -26.584699)
  line L191 (-34.974928, -26.584699) -> (-39.974928, -26.584699)
  line L192 (-39.974928, -26.242007) -> (-39.974928, -23.372477)
  line L193 (-39.974928, -23.372477) -> (-39.186324, -23.372477)
  line L194 (-39.186324, -23.372477) -> (-39.186324, -26.242007)
  line L195 (-39.186324, -26.242007) -> (-39.974928, -26.242007)
  line L196 (-37.807298, -26.242007) -> (-37.807298, -23.7482)
  line L197 (-37.807298, -23.7482) -> (-37.022822, -23.7482)
  line L198 (-37.022822, -23.7482) -> (-37.022822, -26.242007)
  line L199 (-37.022822, -26.242007) -> (-37.807298, -26.242007)
  spline S50 degree 2 poles (-34.925382, -20.957118) (-34.925382, -21.489736) (-35.379552, -22.303113) (-36.217703, -22.749026) (-36.766836, -22.749026) knots 0 0 0 1 2 3 3 3
  line L200 (-36.766836, -22.749026) -> (-38.183021, -22.749026)
  spline S51 degree 2 poles (-38.183021, -22.749026) (-38.732154, -22.749026) (-39.570304, -22.303113) (-40.028603, -21.489736) (-40.028603, -20.957118) knots 0 0 0 1 2 3 3 3
  spline S52 degree 2 poles (-40.028603, -20.957118) (-40.028603, -20.4245) (-39.570304, -19.611123) (-38.732154, -19.165211) (-38.183021, -19.165211) knots 0 0 0 1 2 3 3 3
  line L201 (-38.183021, -19.165211) -> (-36.766836, -19.165211)
  spline S53 degree 2 poles (-36.766836, -19.165211) (-36.217703, -19.165211) (-35.379552, -19.611123) (-34.925382, -20.4245) (-34.925382, -20.957118) knots 0 0 0 1 2 3 3 3
  spline S54 degree 2 poles (-35.742888, -20.957118) (-35.742888, -20.676358) (-35.990618, -20.246961) (-36.444788, -20.011618) (-36.742063, -20.011618) knots 0 0 0 1 2 3 3 3
  line L202 (-36.742063, -20.011618) -> (-38.207794, -20.011618)
  spline S55 degree 2 poles (-38.207794, -20.011618) (-38.509197, -20.011618) (-38.963367, -20.246961) (-39.211097, -20.676358) (-39.211097, -20.957118) knots 0 0 0 1 2 3 3 3
  spline S56 degree 2 poles (-39.211097, -20.957118) (-39.211097, -21.242007) (-38.963367, -21.667275) (-38.509197, -21.902618) (-38.207794, -21.902618) knots 0 0 0 1 2 3 3 3
  line L203 (-38.207794, -21.902618) -> (-36.742063, -21.902618)
  spline S57 degree 2 poles (-36.742063, -21.902618) (-36.444788, -21.902618) (-35.990618, -21.667275) (-35.742888, -21.242007) (-35.742888, -20.957118) knots 0 0 0 1 2 3 3 3
  line L204 (-39.974928, -18.099975) -> (-39.974928, -17.27834)
  line L205 (-39.974928, -17.27834) -> (-34.974928, -17.27834)
  line L206 (-34.974928, -17.27834) -> (-34.974928, -18.099975)
  line L207 (-34.974928, -18.099975) -> (-39.974928, -18.099975)
  line L208 (-35.763533, -17.715995) -> (-35.763533, -14.821693)
  line L209 (-35.763533, -14.821693) -> (-34.974928, -14.821693)
  line L210 (-34.974928, -14.821693) -> (-34.974928, -17.715995)
  line L211 (-34.974928, -17.715995) -> (-35.763533, -17.715995)
  line L212 (-39.974928, -14.06199) -> (-39.974928, -13.240355)
  line L213 (-39.974928, -13.240355) -> (-34.974928, -13.240355)
  line L214 (-34.974928, -13.240355) -> (-34.974928, -14.06199)
  line L215 (-34.974928, -14.06199) -> (-39.974928, -14.06199)
  line L216 (-35.763533, -13.67801) -> (-35.763533, -10.783708)
  line L217 (-35.763533, -10.783708) -> (-34.974928, -10.783708)
  line L218 (-34.974928, -10.783708) -> (-34.974928, -13.67801)
  line L219 (-34.974928, -13.67801) -> (-35.763533, -13.67801)
  spline S58 degree 2 poles (-34.925382, -8.335318) (-34.925382, -8.867936) (-35.379552, -9.681313) (-36.217703, -10.127225) (-36.766836, -10.127225) knots 0 0 0 1 2 3 3 3
  line L220 (-36.766836, -10.127225) -> (-38.183021, -10.127225)
  spline S59 degree 2 poles (-38.183021, -10.127225) (-38.732154, -10.127225) (-39.570304, -9.681313) (-40.028603, -8.867936) (-40.028603, -8.335318) knots 0 0 0 1 2 3 3 3
  spline S60 degree 2 poles (-40.028603, -8.335318) (-40.028603, -7.8027) (-39.570304, -6.989323) (-38.732154, -6.54341) (-38.183021, -6.54341) knots 0 0 0 1 2 3 3 3
  line L221 (-38.183021, -6.54341) -> (-36.766836, -6.54341)
  spline S61 degree 2 poles (-36.766836, -6.54341) (-36.217703, -6.54341) (-35.379552, -6.989323) (-34.925382, -7.8027) (-34.925382, -8.335318) knots 0 0 0 1 2 3 3 3
  spline S62 degree 2 poles (-35.742888, -8.335318) (-35.742888, -8.054558) (-35.990618, -7.625161) (-36.444788, -7.389818) (-36.742063, -7.389818) knots 0 0 0 1 2 3 3 3
  line L222 (-36.742063, -7.389818) -> (-38.207794, -7.389818)
  spline S63 degree 2 poles (-38.207794, -7.389818) (-38.509197, -7.389818) (-38.963367, -7.625161) (-39.211097, -8.054558) (-39.211097, -8.335318) knots 0 0 0 1 2 3 3 3
  spline S64 degree 2 poles (-39.211097, -8.335318) (-39.211097, -8.620206) (-38.963367, -9.045475) (-38.509197, -9.280818) (-38.207794, -9.280818) knots 0 0 0 1 2 3 3 3
  line L223 (-38.207794, -9.280818) -> (-36.742063, -9.280818)
  spline S65 degree 2 poles (-36.742063, -9.280818) (-36.444788, -9.280818) (-35.990618, -9.045475) (-35.742888, -8.620206) (-35.742888, -8.335318) knots 0 0 0 1 2 3 3 3
  line L224 (-39.974928, -3.393121) -> (-39.974928, -2.773799)
  line L225 (-39.974928, -2.773799) -> (-36.345696, -1.782882)
  line L226 (-36.345696, -1.782882) -> (-39.974928, -1.01905)
  line L227 (-39.974928, -1.01905) -> (-39.974928, -0.168514)
  line L228 (-39.974928, -0.168514) -> (-34.974928, -1.357614)
  line L229 (-34.974928, -1.357614) -> (-34.974928, -2.158604)
  line L230 (-34.974928, -2.158604) -> (-38.467909, -3.062816)
  line L231 (-38.467909, -3.062816) -> (-34.974928, -4.008315)
  line L232 (-34.974928, -4.008315) -> (-34.974928, -4.809306)
  line L233 (-34.974928, -4.809306) -> (-39.974928, -5.994277)
  line L234 (-39.974928, -5.994277) -> (-39.974928, -5.14787)
  line L235 (-39.974928, -5.14787) -> (-36.345696, -4.384038)
  line L236 (-36.345696, -4.384038) -> (-39.974928, -3.393121)
  line L237 (-39.974928, 0.487969) -> (-39.974928, 1.309604)
  line L238 (-39.974928, 1.309604) -> (-34.974928, 1.309604)
  line L239 (-34.974928, 1.309604) -> (-34.974928, 0.487969)
  line L240 (-34.974928, 0.487969) -> (-39.974928, 0.487969)
  line L241 (-39.974928, 0.826532) -> (-39.974928, 3.766251)
  line L242 (-39.974928, 3.766251) -> (-39.186324, 3.766251)
  line L243 (-39.186324, 3.766251) -> (-39.186324, 0.826532)
  line L244 (-39.186324, 0.826532) -> (-39.974928, 0.826532)
  line L245 (-35.763533, 0.826532) -> (-35.763533, 3.766251)
  line L246 (-35.763533, 3.766251) -> (-34.974928, 3.766251)
  line L247 (-34.974928, 3.766251) -> (-34.974928, 0.826532)
  line L248 (-34.974928, 0.826532) -> (-35.763533, 0.826532)
  line L249 (-37.852715, 0.826532) -> (-37.852715, 3.390528)
  line L250 (-37.852715, 3.390528) -> (-37.064111, 3.390528)
  line L251 (-37.064111, 3.390528) -> (-37.064111, 0.826532)
  line L252 (-37.064111, 0.826532) -> (-37.852715, 0.826532)
  line L253 (-37.827942, 5.037927) -> (-37.827942, 6.759645)
  spline S66 degree 2 poles (-37.827942, 6.759645) (-37.827942, 6.933055) (-37.993095, 7.1973) (-38.306885, 7.341808) (-38.509197, 7.345937) knots 0 0 0 1 2 3 3 3
  spline S67 degree 2 poles (-38.509197, 7.345937) (-38.711509, 7.345937) (-39.021171, 7.201429) (-39.190452, 6.937184) (-39.190452, 6.759645) knots 0 0 0 1 2 3 3 3
  line L254 (-39.190452, 6.759645) -> (-39.190452, 5.037927)
  line L255 (-39.190452, 5.037927) -> (-39.979057, 5.037927)
  line L256 (-39.979057, 5.037927) -> (-39.979057, 6.784418)
  spline S68 degree 2 poles (-39.979057, 6.784418) (-39.979057, 7.209686) (-39.615721, 7.849653) (-38.946852, 8.200603) (-38.509197, 8.200603) knots 0 0 0 1 2 3 3 3
  spline S69 degree 2 poles (-38.509197, 8.200603) (-38.071542, 8.200603) (-37.402674, 7.849653) (-37.039338, 7.205557) (-37.039338, 6.784418) knots 0 0 0 1 2 3 3 3
  line L257 (-37.039338, 6.784418) -> (-37.039338, 5.037927)
  line L258 (-37.039338, 5.037927) -> (-37.827942, 5.037927)
  line L259 (-39.979057, 4.699364) -> (-39.979057, 5.520999)
  line L260 (-39.979057, 5.520999) -> (-34.974928, 5.520999)
  line L261 (-34.974928, 5.520999) -> (-34.974928, 4.699364)
  line L262 (-34.974928, 4.699364) -> (-39.979057, 4.699364)
  line L263 (-37.192104, 6.243543) -> (-37.353128, 7.098208)
  line L264 (-37.353128, 7.098208) -> (-34.974928, 8.411173)
  line L265 (-34.974928, 8.411173) -> (-34.974928, 7.424385)
  line L266 (-34.974928, 7.424385) -> (-37.192104, 6.243543)
  line L267 (-39.974928, 11.18161) -> (-39.974928, 12.003245)
  line L268 (-39.974928, 12.003245) -> (-34.974928, 12.003245)
  line L269 (-34.974928, 12.003245) -> (-34.974928, 11.18161)
  line L270 (-34.974928, 11.18161) -> (-39.974928, 11.18161)
  line L271 (-35.763533, 11.56559) -> (-35.763533, 14.459893)
  line L272 (-35.763533, 14.459893) -> (-34.974928, 14.459893)
  line L273 (-34.974928, 14.459893) -> (-34.974928, 11.56559)
  line L274 (-34.974928, 11.56559) -> (-35.763533, 11.56559)
  line L275 (-39.974928, 16.615136) -> (-39.974928, 17.213815)
  line L276 (-39.974928, 17.213815) -> (-34.974928, 19.092428)
  line L277 (-34.974928, 19.092428) -> (-34.974928, 18.20886)
  line L278 (-34.974928, 18.20886) -> (-38.699123, 16.912411)
  line L279 (-38.699123, 16.912411) -> (-34.974928, 15.62422)
  line L280 (-34.974928, 15.62422) -> (-34.974928, 14.736524)
  line L281 (-34.974928, 14.736524) -> (-39.974928, 16.615136)
  line L282 (-36.713161, 15.620091) -> (-36.713161, 18.250149)
  line L283 (-36.713161, 18.250149) -> (-35.924557, 18.250149)
  line L284 (-35.924557, 18.250149) -> (-35.924557, 15.620091)
  line L285 (-35.924557, 15.620091) -> (-36.713161, 15.620091)
  line L286 (-37.704078, 20.174178) -> (-37.704078, 21.77616)
  spline S70 degree 2 poles (-37.704078, 21.77616) (-37.704078, 21.974344) (-37.889874, 22.275747) (-38.224309, 22.4409) (-38.443136, 22.4409) knots 0 0 0 1 2 3 3 3
  spline S71 degree 2 poles (-38.443136, 22.4409) (-38.666092, 22.4409) (-39.000527, 22.275747) (-39.186324, 21.974344) (-39.186324, 21.77616) knots 0 0 0 1 2 3 3 3
  line L287 (-39.186324, 21.77616) -> (-39.186324, 20.174178)
  line L288 (-39.186324, 20.174178) -> (-39.974928, 20.174178)
  line L289 (-39.974928, 20.174178) -> (-39.974928, 21.751387)
  spline S72 degree 2 poles (-39.974928, 21.751387) (-39.974928, 22.209686) (-39.595077, 22.907457) (-38.897306, 23.287308) (-38.443136, 23.287308) knots 0 0 0 1 2 3 3 3
  spline S73 degree 2 poles (-38.443136, 23.287308) (-37.984837, 23.287308) (-37.291196, 22.907457) (-36.915473, 22.209686) (-36.915473, 21.751387) knots 0 0 0 1 2 3 3 3
  line L290 (-36.915473, 21.751387) -> (-36.915473, 20.174178)
  line L291 (-36.915473, 20.174178) -> (-37.704078, 20.174178)
  line L292 (-39.974928, 19.781941) -> (-39.974928, 20.603576)
  line L293 (-39.974928, 20.603576) -> (-34.974928, 20.603576)
  line L294 (-34.974928, 20.603576) -> (-34.974928, 19.781941)
  line L295 (-34.974928, 19.781941) -> (-39.974928, 19.781941)
  line L296 (-39.566175, 26.759645) -> (-39.566175, 27.58128)
  line L297 (-39.566175, 27.58128) -> (-34.974928, 27.58128)
  line L298 (-34.974928, 27.58128) -> (-34.974928, 26.759645)
  line L299 (-34.974928, 26.759645) -> (-39.566175, 26.759645)
  line L300 (-39.974928, 25.368233) -> (-39.974928, 28.964434)
  line L301 (-39.974928, 28.964434) -> (-39.186324, 28.964434)
  line L302 (-39.186324, 28.964434) -> (-39.186324, 25.368233)
  line L303 (-39.186324, 25.368233) -> (-39.974928, 25.368233)
  line L304 (-34.974928, 30.256755) -> (-34.974928, 29.414476)
  line L305 (-34.974928, 29.414476) -> (-39.974928, 29.414476)
  line L306 (-39.974928, 29.414476) -> (-39.974928, 30.256755)
  line L307 (-39.974928, 30.256755) -> (-34.974928, 30.256755)
  line L308 (-34.904912, 35.175741) -> (-34.904912, 34.607372)
  line L309 (-34.904912, 34.607372) -> (-38.743462, 34.607372)
  line L310 (-38.743462, 34.607372) -> (-36.115785, 33.293534)
  line L311 (-36.115785, 33.293534) -> (-38.743462, 31.979695)
  line L312 (-38.743462, 31.979695) -> (-34.904912, 31.979695)
  line L313 (-34.904912, 31.979695) -> (-34.904912, 31.411326)
  line L314 (-34.904912, 31.411326) -> (-39.904912, 31.411326)
  line L315 (-39.904912, 31.411326) -> (-39.904912, 31.897323)
  line L316 (-39.904912, 31.897323) -> (-37.170151, 33.293534)
  line L317 (-37.170151, 33.293534) -> (-39.904912, 34.689745)
  line L318 (-39.904912, 34.689745) -> (-39.904912, 35.175741)
  line L319 (-39.904912, 35.175741) -> (-34.904912, 35.175741)
  line L320 (-39.974928, 36.231556) -> (-39.974928, 37.053191)
  line L321 (-39.974928, 37.053191) -> (-34.974928, 37.053191)
  line L322 (-34.974928, 37.053191) -> (-34.974928, 36.231556)
  line L323 (-34.974928, 36.231556) -> (-39.974928, 36.231556)
  line L324 (-39.974928, 36.570119) -> (-39.974928, 39.509838)
  line L325 (-39.974928, 39.509838) -> (-39.186324, 39.509838)
  line L326 (-39.186324, 39.509838) -> (-39.186324, 36.570119)
  line L327 (-39.186324, 36.570119) -> (-39.974928, 36.570119)
  line L328 (-35.763533, 36.570119) -> (-35.763533, 39.509838)
  line L329 (-35.763533, 39.509838) -> (-34.974928, 39.509838)
  line L330 (-34.974928, 39.509838) -> (-34.974928, 36.570119)
  line L331 (-34.974928, 36.570119) -> (-35.763533, 36.570119)
  line L332 (-37.852715, 36.570119) -> (-37.852715, 39.134116)
  line L333 (-37.852715, 39.134116) -> (-37.064111, 39.134116)
  line L334 (-37.064111, 39.134116) -> (-37.064111, 36.570119)
  line L335 (-37.064111, 36.570119) -> (-37.852715, 36.570119)
  line L336 (-37.827942, 40.781514) -> (-37.827942, 42.503232)
  spline S74 degree 2 poles (-37.827942, 42.503232) (-37.827942, 42.676642) (-37.993095, 42.940887) (-38.306885, 43.085395) (-38.509197, 43.089524) knots 0 0 0 1 2 3 3 3
  spline S75 degree 2 poles (-38.509197, 43.089524) (-38.711509, 43.089524) (-39.021171, 42.945016) (-39.190452, 42.680771) (-39.190452, 42.503232) knots 0 0 0 1 2 3 3 3
  line L337 (-39.190452, 42.503232) -> (-39.190452, 40.781514)
  line L338 (-39.190452, 40.781514) -> (-39.979057, 40.781514)
  line L339 (-39.979057, 40.781514) -> (-39.979057, 42.528005)
  spline S76 degree 2 poles (-39.979057, 42.528005) (-39.979057, 42.953273) (-39.615721, 43.59324) (-38.946852, 43.94419) (-38.509197, 43.94419) knots 0 0 0 1 2 3 3 3
  spline S77 degree 2 poles (-38.509197, 43.94419) (-38.071542, 43.94419) (-37.402674, 43.59324) (-37.039338, 42.949144) (-37.039338, 42.528005) knots 0 0 0 1 2 3 3 3
  line L340 (-37.039338, 42.528005) -> (-37.039338, 40.781514)
  line L341 (-37.039338, 40.781514) -> (-37.827942, 40.781514)
  line L342 (-39.979057, 40.442951) -> (-39.979057, 41.264586)
  line L343 (-39.979057, 41.264586) -> (-34.974928, 41.264586)
  line L344 (-34.974928, 41.264586) -> (-34.974928, 40.442951)
  line L345 (-34.974928, 40.442951) -> (-39.979057, 40.442951)
  line L346 (-37.192104, 41.98713) -> (-37.353128, 42.841795)
  line L347 (-37.353128, 42.841795) -> (-34.974928, 44.15476)
  line L348 (-34.974928, 44.15476) -> (-34.974928, 43.167972)
  line L349 (-34.974928, 43.167972) -> (-37.192104, 41.98713)
  point P0 (0, 0)
  point P1 (5, -22.682965)
  point P2 (5, 8.753762)
  point P3 (5, 40.714039)
  point P4 (6.470983, -30)
  point P5 (6.470983, 0)
  point P6 (6.470983, 30)
  point P7 (-40.028603, 0)
  point P8 (-43.3, 0)
  dimension "d81" = 20
  constraints: 8 midpoint, 4 horizontal alignment, 2 vertical alignment, 8 other
  measures "d81" horizontal distance of A0.centre point (5, -22.683)